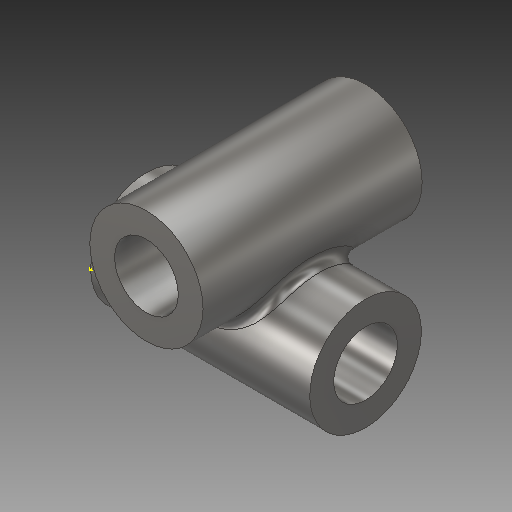
# Autodesk Inventor part: Centre Block
Saved by Autodesk Inventor 2018 (Build 220112000, 112)
## iProperties
Created: 2018-09-13
Part Number: Centre Block
Material: Stainless Steel
Document SubType Name: Modeling
Designer: Ajay Sharma
Density: 8 g/cm^3
Appearance: Semi-Polished
Author: Ajay Sharma
Autodesk Inventor part; units mm, degrees
ref_plane "YZ Plane" through (0, 0, 0) normal (1, 0, 0) x (0, 1, 0)
ref_plane "XZ Plane" through (0, 0, 0) normal (0, 1, 0) x (-1, 0, 0)
sketch "Sketch1" plane through (0, 0, 0) normal (1, 0, 0) x (0, 1, 0)
  line L0 (-39.2, 0) -> (39.2, 0) projected
  line L1 (0, 39.2) -> (0, -39.2) projected
  circle A0 centre (0, 0) radius 28
  circle A1 centre (0, 0) radius 16
  dimension "d0" = 56
  dimension "d1" = 32
  constraints: 2 centre point, 2 coincident
  measures "d0" diameter of A0
  measures "d1" diameter of A1
extrude "Extrusion1" add sketch "Sketch1" along normal blind 110 contours A1 L1 A0 L0 | L0 A0 L1 A1 | A1 L0 A0 L1 | L1 A0 L0 A1
ref_plane "Work Plane1" through (0, 0, 28) normal (0, 0, 1) x (1, 0, 0)
sketch "Sketch2" plane through (0, 0, 28) normal (0, 0, 1) x (1, 0, 0)
  line L0 (-22, 0) -> (132, 0) projected
  circle A0 centre (55, 38) radius 28.4253
  circle A1 centre (55, 38) radius 16
  point P0 (0, 0)
  dimension "d6" = 32
  constraints: 2 centre point, 1 coincident
  measures "d6" diameter of A1
extrude "Extrusion2" add sketch "Sketch2" along normal blind 27 and the other way blind 83
sketch "Sketch3" plane through (0, 0, 28) normal (0, 0, 1) x (1, 0, 0)
  point P0 (0, 0)
fillet "Fillet1" radius 4 2 edges at (55, 9.5747, -26.3121) (55, 9.5747, 26.3121)
sketch "Sketch4" plane through (110, 0, 0) normal (1, 0, 0) x (0, 0, -1)
  circle A0 centre (0, 0) radius 16
  constraints: 1 centre point, 1 coincident
extrude "Extrusion3" cut sketch "Sketch4" against normal through all
sketch "Sketch5" plane through (55, 38, 55) normal (0, 0, 1) x (1, 0, 0)
  circle A0 centre (0, 0) radius 16
  point P0 (-55, -38)
  constraints: 1 centre point
extrude "Extrusion4" cut sketch "Sketch5" against normal through all
body "Solid1"
